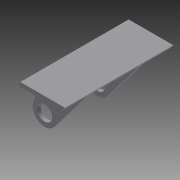
# Autodesk Inventor part: Head_v2
Saved by Autodesk Inventor 2013 (Build 170138000, 138)
## iProperties
Created: 2012-11-28
Part Number: Head_v2
Material: Generic
Document SubType Name: Modeling
Designer: Joe
Density: 1 g/cm^3
Author: Joe
Autodesk Inventor part; units mm, degrees
ref_plane "YZ Plane" through (0, 0, 0) normal (1, 0, 0) x (0, 1, 0)
ref_plane "XZ Plane" through (0, 0, 0) normal (0, 1, 0) x (-1, 0, 0)
sketch "Sketch1" plane through (0, 0, 0) normal (1, 0, 0) x (0, 1, 0)
  circle A0 centre (0, 0) radius 10
  arc A1 (-9.7398, 12.694) -> (5.3275, -15.087) centre (0, 0) ccw
  line L0 (0, 0) -> (0, 61.6) construction
  line L1 (0, 0) -> (54, 0) construction
  line L2 (0, 61.6) -> (54, 61.6) construction
  line L3 (54, 0) -> (54, 61.6) construction
  line L4 (54, 61.6) -> (54, 2.1)
  line L5 (54, 61.6) -> (-9.7398, 12.694)
  line L6 (54, 2.1) -> (5.3275, -15.087)
  dimension "d0" = 20
  dimension "d2" = 32
  dimension "d3" = 61.6
  dimension "d4" = 54
  dimension "d5" = 59.5
  constraints: 14 end point, 2 centre point, 2 coincident, 2 perpendicular, 2 point on circle, 2 tangent, 1 parallel, 1 point on line, 1 vertical
  measures "d0" diameter of A0
  measures "d2" diameter of A1
  measures "d3" distance of L0.start L0.end
  measures "d4" distance of L0.start L1.end
  measures "d5" distance of L2.end L4.end
extrude "Extrusion1" add sketch "Sketch1" along normal blind 144.45
sketch "Sketch2" plane through (0, 0, 0) normal (0, 0, 1) x (1, 0, 0)
  line L0 (0, 54) -> (144.45, 54) projected
  line L1 (0, -9.7398) -> (0, 54) projected
  line L2 (0, -9.7398) -> (144.45, -9.7398) projected
  line L3 (144.45, 54) -> (144.45, -9.7398) projected
  line L4 (0, 54) -> (144.45, 54) projected
  line L5 (72.225, 54) -> (72.225, -21.6932)
  line L6 (39.225, 48) -> (105.225, 48)
  line L7 (105.225, 48) -> (105.225, -39.8615)
  line L8 (105.225, -39.8615) -> (39.225, -39.8615)
  line L9 (39.225, -39.8615) -> (39.225, 48)
  line L10 (72.225, 48) -> (72.225, -39.8615)
  point P0 (0, 0)
  dimension "d8" = 66
  dimension "d10" = 6
  constraints: 12 end point, 3 midpoint, 2 parallel, 2 perpendicular, 1 collinear, 1 horizontal
  measures "d8" distance of L7.end L8.end
  measures "d10" distance between parallel lines of L6 L0
extrude "Extrusion2" cut sketch "Sketch2" along normal mid plane 144.45 contours L6 L7 L2 L5 | L5 L2 L9 L6 | L2 L5 L10 L8 L9 | L2 L7 L8 L10 L5
ref_plane "Work Plane1" through (72.225, 0, 0) normal (1, 0, 0) x (0, 0, -1)
sketch "Sketch3" plane through (0, 0, 0) normal (0, 0, 1) x (1, 0, 0)
  line L0 (0, 54) -> (144.45, 54) projected
  line L1 (144.45, 54) -> (144.45, -9.7398) projected
  line L2 (105.225, 48) -> (105.225, -9.7398) projected
  line L3 (105.225, -9.7398) -> (144.45, -9.7398) projected
  line L4 (144.45, 54) -> (144.45, -9.7398) projected
  line L5 (0, 54) -> (144.45, 54) projected
  line L6 (0, -9.7398) -> (0, 54) projected
  line L7 (0, -9.7398) -> (39.225, -9.7398) projected
  line L8 (39.225, -9.7398) -> (39.225, 48) projected
  line L9 (39.225, 48) -> (105.225, 48) projected
  line L10 (144.45, 48) -> (109.925, 48)
  line L11 (109.925, 48) -> (109.925, -25.7164)
  line L12 (109.925, -25.7164) -> (144.45, -25.7164)
  line L13 (144.45, -25.7164) -> (144.45, 48)
  line L14 (39.225, 48) -> (105.225, 48) projected
  point P0 (0, 0)
  dimension "d14" = 34.525
  constraints: 8 end point, 2 collinear, 2 parallel, 1 horizontal, 1 perpendicular
  measures "d14" distance of L11.end L12.end
extrude "Extrusion3" cut sketch "Sketch3" along normal through all both and the other way through all contours L1 L3 L11 L10 | L13 L12 L11 L3
mirror "Mirror1" about plane through (72.225, 0, 0) normal (1, 0, 0) of "Extrusion3"
move or copy body "Move Body1" bodies to move or copy 1 copy no translate (-72.225, 0, 0)
move or copy body "Move Body2" bodies to move or copy 1 copy no rotation origin (0, 0, 0) rotation axis (1, 0, 0) rotation angle 90
move or copy body "Move Body4" bodies to move or copy 1 copy no rotation origin (0, 0, 0) rotation axis (0, 0, 1) rotation angle 90
body "Solid1"
